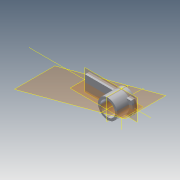
# Autodesk Inventor part: HbThumbProximalPhalanxBase01
Saved by Autodesk Inventor 2015 SP1 (Build 190203100, 203)
## iProperties
Created: 2015-09-12
Part Number: HbThumbProximalPhalanxBase01
Material: ABS プラスチック
Document SubType Name: Modeling
Designer: Yamaura
Density: 1.06 g/cm^3
Appearance: 滑らか - 白
Author: Yamaura
Autodesk Inventor part; units mm, degrees
sketch "スケッチ1" plane through (0, 0, 0) normal (0, 0, 1) x (1, 0, 0)
  circle A0 centre (0, 0) radius 5.25
  circle A1 centre (0, 0) radius 7.05
  dimension "d0" = 10.5
  dimension "d1" = 14.1
  constraints: 2 centre point, 2 coincident
  measures "d0" diameter of A0
  measures "d1" diameter of A1
extrude "押し出し1" add sketch "スケッチ1" along normal blind 10 and the other way blind 3.5 contours A0 | A1
sketch "スケッチ2" plane through (0, 0, 0) normal (0, 0, 1) x (1, 0, 0)
  line L0 (-25, 5) -> (0, 5)
  line L1 (0, 5) -> (0, -5)
  line L2 (0, -5) -> (-25, -5)
  line L3 (-25, -5) -> (-25, 5)
  point P0 (0, 0)
  dimension "d4" = 25
  dimension "d5" = 5
  dimension "d6" = 10
  constraints: 8 end point, 2 parallel, 1 horizontal, 1 midpoint, 1 perpendicular
  measures "d4" distance from line of L3 point (0, 0)
  measures "d5" distance from line of L0 point (0, 0)
  measures "d6" distance of L2.end L0.start
extrude "押し出し2" add sketch "スケッチ2" along normal mid plane 3
sketch "スケッチ5" plane through (0, 0, -3.5) normal (0, 0, -1) x (-1, 0, 0)
  circle A0 centre (0, 0) radius 5.35
  dimension "d21" = 10.7
  constraints: 1 centre point, 1 coincident
  measures "d21" diameter of A0
extrude "押し出し5" cut sketch "スケッチ5" against normal through all
sketch "スケッチ9" plane through (0, 0, 0) normal (0, 0, 1) x (1, 0, 0)
  line L0 (8.4285, -5) -> (-7.6033, -5)
  line L1 (-7.6033, 5) -> (8.4285, 5)
  arc A0 (4.9702, -5) -> (4.9702, 5) centre (0, 0) ccw
  arc A1 (-4.9702, 5) -> (-4.9702, -5) centre (0, 0) ccw
  arc A2 (8.4285, -5) -> (8.4285, 5) centre (0, 0) ccw
  arc A3 (-7.6033, 5) -> (-7.6033, -5) centre (0, 0) ccw
  dimension "d74" = 5
  dimension "d75" = 5
  dimension "d79" = 9.8
  constraints: 8 point on circle, 4 centre point, 4 end point, 4 point on line, 2 coincident, 1 horizontal, 1 parallel
  measures "d74" distance from line of L0 point (0, 0)
  measures "d75" distance from line of L1 point (0, 0)
  measures "d79" radius of A2
extrude "押し出し9" add sketch "スケッチ9" along normal mid plane 3 contours L0 A0 L1 A2
sketch "スケッチ6" plane through (0, 0, -3.5) normal (0, 0, -1) x (-1, 0, 0)
  line L0 (7.2132, -2.9681) -> (-7.7309, 1.0362)
  line L1 (-7.2132, 2.9681) -> (7.7309, -1.0362)
  line L2 (11.6181, 0) -> (-15.1574, 0) projected
  arc A0 (7.2132, -2.9681) -> (7.7309, -1.0362) centre (0, 0) ccw
  arc A1 (-7.2132, 2.9681) -> (-7.7309, 1.0362) centre (0, 0) ccw
  point P0 (-11.3323, 4.0718)
  dimension "d24" = 1
  dimension "d43" = 15
  dimension "d64" = 1
  dimension "d65" = 7.8
  dimension "d66" = 7.8
  constraints: 4 end point, 4 point on circle, 2 centre point, 1 coincident, 1 parallel
  measures "d24" distance from line of L0 point (0, 0)
  measures "d43" angle of L0 L2
  measures "d64" distance from line of L1 point (0, 0)
  measures "d65" radius of A0
  measures "d66" radius of A1
extrude "押し出し6" cut sketch "スケッチ6" against normal blind 3.5
pattern_circular "円形状パターン2" count 2 over 30 about axis through (0, 0, -10) along (0, 0, -1) of "押し出し6"
move faces "移動4" translate (0, 0, 2) faces at (-6.4599, -0.5051, -3.5) (6.4791, 0.0439, -3.5)
ref_plane "作業平面1" through (0, 0, 0) normal (-0.258819, 0.9659258, 0) x (0, 0, 1)
chamfer "面取り1" distance 0.5 angle 45 4 edges at (-7.7309, 1.0362, -0.75) (-7.7309, -1.0362, -0.75) (7.7309, -1.0362, -0.75) (7.7309, 1.0362, -0.75)
